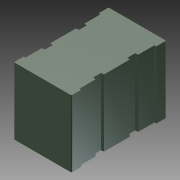
# Autodesk Inventor part: M20111SS1W01-switch
Saved by Autodesk Inventor 2015 SP1 (Build 190203100, 203)
## iProperties
Category: PARTsolutions
Company: NKKSWITCHES
Created: 2013-12-29
Part Number: M20111SS1W01-switch
Catalog Web Link: www.cadenas.de
Description: Bushing Mount Miniature Toggles - Switch-Series M - Miniature Toggles
Vendor: NKKSWITCHES
Document SubType Name: Modeling
Designer: PARTuser1
Manufacturer: NKKSWITCHES
Density: 1 g/cm^3
Material: Generic
Appearance: RGB(78.00000295042994,110.00000104308060,71.00000336766270)
PSOL_IDENT_0: {$CADENAS_DATA\23d-libs\nkkswitches\toggle\m\parts\m_bt_switch.prj},260 {VTYP=3D},{NB=M20111SS1W01-s
PSOL_IDENT_1: witch},{LINA=M20111SS1W01-switch},{NN=Bushing Mount Miniature Toggles - Switch},{DATE=28.05.2013 10:
PSOL_IDENT_2: 56:01},{GEOMDATE=28.05.2013 12:19:00},{VERSION=},{LINEID=10},{LINESUBID=-1},{WBVAR=PLS,CRCTS,TGGL,TG
PSOL_IDENT_3: GLS,BSHNG,CMR,TRMNLS,CPS,CCLR}  {NB=M20111SS1W01-switch},{LINA=M20111SS1W01-switch},{KT=DUMMY},{PN=M
PSOL_IDENT_4: 20111SS1W01},{SRS=M20},{PLS=1},{CRCTSALG='1','1 - ON/NONE/OFF','2','2 - ON/NONE/ON','3','3 - ON/OFF/
PSOL_IDENT_5: ON','5','5 - ON/NONE/(ON)','8','8 - (ON)/OFF/(ON)','9','9 - ON/OFF/(ON)','4', '4 - ON/ON/ON','6','6
PSOL_IDENT_6: - (ON)/ON/(ON)','7','7 - ON/ON/(ON)'},{CRCTS=1},{TGGL=1},{TGGLSALG='S', 'S - .413\" (10.5mm) Bat','S
PSOL_IDENT_7: 2', 'S2 - .200\" (5.08mm) Bat','S3', 'S3 - .256\" (6.5mm) Bat','E', 'E - .450\" (11.4mm) Flatted','E
PSOL_IDENT_8: 2', 'E2 - .256\" (6.5mm) Flatted','E4', 'E4 - .840\" (21.3mm) Flatted','Q', 'Q - .550\" (14.0mm) Con
PSOL_IDENT_9: e','Q2', 'Q2 - .640\" (16.26mm) Cone','Q4', 'Q4 - .840\" (21.3mm) Cone','C', 'C - .571\" (14.5mm) Co
PSOL_IDENT_10: lor Tipped Cone','D', 'D - .840\" (21.3mm) Color Tipped Cone','K1', 'K1 - .370\" (9.4mm) Paddle','K2
PSOL_IDENT_11: ', 'K2 - .559\" (14.2mm) Paddle'},{TGGLS=S},{BSHNGALG='S1', 'S1 - .350\" (8.9mm) Threaded with Keywa
PSOL_IDENT_12: y','S2', 'S2 - .350\" (8.9mm) Smooth with Keyway','A1', 'A1 - .280\" (7.1mm) Threaded with Keyway','
PSOL_IDENT_13: A2', 'A2 - .280\" (7.1mm) Smooth with Keyway','D1', 'D1 - .350\" (8.9mm) Threaded with D Flat','D4'
PSOL_IDENT_14: , 'D4 - 6mm .350\" (8.9mm) Threaded with D Flat ' ,'D3', 'D3 - .350\" (8.9mm) Threaded Splashproof w
PSOL_IDENT_15: ith D Flat','S4', 'S4 - 6mm .350\" (8.9mm) Threaded with Keyway','D8', 'D8 - 6mm .350\" (8.9mm) Thre
PSOL_IDENT_16: aded Splashproof with D Flat'},{BSHNG=S1},{CMR=W},{TRMNLSALG='01','01 - Solder Lug','02','02 - Quick
PSOL_IDENT_17: Connect','03','03 - .250\" (6.35mm) Straight PC','05', '05 - .425\" (10.8mm) Wirewrap','06', '06 -
PSOL_IDENT_18: .750\" (19.05mm) Wirewrap','07', '07 - .964\" (24.5mm) Wirewrap','08', '08 - 1.062\" (27.0mm) Wirewr
PSOL_IDENT_19: ap'},{TRMNLS=01},{CPSALG='','w/o Cap','B', 'B - For S Bat Toggle','C', 'C - Conical Cap for S Bat To
PSOL_IDENT_20: ggle'},{CPS=},{CPSPN=},{CCLRALG='','N/A'},{CCLR=},{DSH=},{WIDTH=0.512},{HEIGHT=0.371},{LENGTH=0.311}
PSOL_IDENT_21: ,{A=0},{TRMNLNOH=1},{ROTALG=0.2625},{ANG=12.5},{TRMNLOV=2},{LTRMNL=0.079},{POS=0}
CNS_NN: Bushing Mount Miniature Toggles - Switch
CNS_NT: Series M - Miniature Toggles
CNS_NB: M20111SS1W01-switch
CNS_NBSYN: $PN.-switch
CNS_LINA: M20111SS1W01-switch
CNS_PN: M20111SS1W01
CNS_SRS: M20
CNS_PLS: 1 - SPST/SPDT
CNS_CRCTSALG: '1','1 - ON/NONE/OFF','2','2 - ON/NONE/ON','3','3 - ON/OFF/ON','5','5 - ON/NONE/(ON)','8','8 - (ON)/OFF/(ON)','9','9 - ON/OFF/(ON)','4', '4 - ON/ON/ON','6','6 - (ON)/ON/(ON)','7','7 - ON/ON/(ON)'
CNS_CRCTS: 1 - ON/NONE/OFF
CNS_TGGL: Small Toggles
CNS_TGGLSALG: 'S', 'S - .413" (10.5mm) Bat','S2', 'S2 - .200" (5.08mm) Bat','S3', 'S3 - .256" (6.5mm) Bat','E', 'E - .450" (11.4mm) Flatted','E2', 'E2 - .256" (6.5mm) Flatted','E4', 'E4 - .840" (21.3mm) Flatted','Q', 'Q - .550" (14.0mm) Cone','Q2', 'Q2 - .640" (16.26mm) Cone','Q4', 'Q4 - .840" (21.3mm) Cone','C', 'C - .571" (14.5mm) Color Tipped Cone','D', 'D - .840" (21.3mm) Color Tipped Cone','K1', 'K1 - .370" (9.4mm) Paddle','K2', 'K2 - .559" (14.2mm) Paddle'
CNS_TGGLS: S - .413" (10.5mm) Bat
CNS_BSHNGALG: 'S1', 'S1 - .350" (8.9mm) Threaded with Keyway','S2', 'S2 - .350" (8.9mm) Smooth with Keyway','A1', 'A1 - .280" (7.1mm) Threaded with Keyway','A2', 'A2 - .280" (7.1mm) Smooth with Keyway','D1', 'D1 - .350" (8.9mm) Threaded with D Flat','D4' , 'D4 - 6mm .350" (8.9mm) Threaded with D Flat ' ,'D3', 'D3 - .350" (8.9mm) Threaded Splashproof with D Flat','S4', 'S4 - 6mm .350" (8.9mm) Threaded with Keyway','D8', 'D8 - 6mm .350" (8.9mm) Threaded Splashproof with D Flat'
CNS_BSHNG: S1 - .350" (8.9mm) Threaded with Keyway
CNS_CMR: W - Silver; Rated 6A @ 125V AC & 3A @ 250V AC
CNS_TRMNLSALG: '01','01 - Solder Lug','02','02 - Quick Connect','03','03 - .250" (6.35mm) Straight PC','05', '05 - .425" (10.8mm) Wirewrap','06', '06 - .750" (19.05mm) Wirewrap','07', '07 - .964" (24.5mm) Wirewrap','08', '08 - 1.062" (27.0mm) Wirewrap'
CNS_TRMNLS: 01 - Solder Lug
CNS_CPSALG: '','w/o Cap','B', 'B - For S Bat Toggle','C', 'C - Conical Cap for S Bat Toggle'
CNS_CPS: w/o Cap
CNS_CCLRALG: '','N/A'
CNS_CCLR: N/A
CNS_WIDTH: 0.512
CNS_HEIGHT: 0.371
CNS_LENGTH: 0.311
CNS_A: 0.000
CNS_TRMNLNOH: 1.000
CNS_ROTALG: 0.262
CNS_ANG: 12.500
CNS_TRMNLOV: 2.000
CNS_LTRMNL: 0.079
CNS_POS: 0.000
SUPPLIER: NKKSWITCHES
ARTICLENO: M20111SS1W01-switch
BOMINFO: M20111SS1W01-switch
CREATOR: CADENAS GmbH
Title: M20111SS1W01-switch
Author: Cadenas PARTsolutions
Comments: Series M - Miniature Toggles
Autodesk Inventor part; units mm, degrees
sketch "Sketch_2" plane through (0, -0.254, 0) normal (0, 1, 0) x (1, 0, 0)
  line L0 (-3.9497, -5.1435) -> (-3.9497, -6.3724)
  arc A0 (-3.9497, -6.3724) -> (-3.8197, -6.5024) centre (-3.8197, -6.3724) ccw
  line L1 (-3.8197, -6.5024) -> (3.8197, -6.5024)
  arc A1 (3.8197, -6.5024) -> (3.9497, -6.3724) centre (3.8197, -6.3724) ccw
  line L2 (3.9497, -6.3724) -> (3.9497, -5.1435)
  line L3 (3.9497, -5.1435) -> (3.6957, -5.1435)
  line L4 (3.6957, -5.1435) -> (3.6957, -2.9397)
  line L5 (3.6957, -2.9397) -> (3.3147, -2.8725)
  line L6 (3.3147, -2.8725) -> (3.3147, -1.8265)
  line L7 (3.3147, -1.8265) -> (3.6957, -1.7593)
  line L8 (3.6957, -1.7593) -> (3.6957, 1.7593)
  line L9 (3.6957, 1.7593) -> (3.3147, 1.8265)
  line L10 (3.3147, 1.8265) -> (3.3147, 2.8725)
  line L11 (3.3147, 2.8725) -> (3.6957, 2.9397)
  line L12 (3.6957, 2.9397) -> (3.6957, 5.1435)
  line L13 (3.6957, 5.1435) -> (3.9497, 5.1435)
  line L14 (3.9497, 5.1435) -> (3.9497, 6.3724)
  arc A2 (3.9497, 6.3724) -> (3.8197, 6.5024) centre (3.8197, 6.3724) ccw
  line L15 (3.8197, 6.5024) -> (-3.8197, 6.5024)
  arc A3 (-3.8197, 6.5024) -> (-3.9497, 6.3724) centre (-3.8197, 6.3724) ccw
  line L16 (-3.9497, 6.3724) -> (-3.9497, 5.1435)
  line L17 (-3.9497, 5.1435) -> (-3.6957, 5.1435)
  line L18 (-3.6957, 5.1435) -> (-3.6957, 2.9397)
  line L19 (-3.6957, 2.9397) -> (-3.3147, 2.8725)
  line L20 (-3.3147, 2.8725) -> (-3.3147, 1.8265)
  line L21 (-3.3147, 1.8265) -> (-3.6957, 1.7593)
  line L22 (-3.6957, 1.7593) -> (-3.6957, -1.7593)
  line L23 (-3.6957, -1.7593) -> (-3.3147, -1.8265)
  line L24 (-3.3147, -1.8265) -> (-3.3147, -2.8725)
  line L25 (-3.3147, -2.8725) -> (-3.6957, -2.9397)
  line L26 (-3.6957, -2.9397) -> (-3.6957, -5.1435)
  line L27 (-3.6957, -5.1435) -> (-3.9497, -5.1435)
  constraints: 56 end point, 8 point on circle, 4 centre point
extrude "Extrusion1" add sketch "Sketch_2" against normal blind 9.1694
sketch "Sketch_1" plane through (0, -9.4234, 0) normal (0, 1, 0) x (1, 0, 0)
  line L0 (-3.1877, 6.1184) -> (-3.1877, -6.1184)
  arc A0 (-3.1877, -6.1184) -> (-3.0577, -6.2484) centre (-3.0577, -6.1184) ccw
  line L1 (-3.0577, -6.2484) -> (3.0577, -6.2484)
  arc A1 (3.0577, -6.2484) -> (3.1877, -6.1184) centre (3.0577, -6.1184) ccw
  line L2 (3.1877, -6.1184) -> (3.1877, 6.1184)
  arc A2 (3.1877, 6.1184) -> (3.0577, 6.2484) centre (3.0577, 6.1184) ccw
  line L3 (3.0577, 6.2484) -> (-3.0577, 6.2484)
  arc A3 (-3.0577, 6.2484) -> (-3.1877, 6.1184) centre (-3.0577, 6.1184) ccw
  constraints: 8 end point, 8 point on circle, 4 centre point
extrude "Extrusion2" cut sketch "Sketch_1" along normal blind 0.0254
sketch "Sketch_7" plane through (0, -9.4234, 0) normal (0, 1, 0) x (1, 0, 0)
  line L0 (-1.0033, 5.0927) -> (-1.0033, 4.3053)
  line L1 (-1.0033, 4.3053) -> (1.0033, 4.3053)
  line L2 (1.0033, 4.3053) -> (1.0033, 5.0927)
  line L3 (1.0033, 5.0927) -> (-1.0033, 5.0927)
  constraints: 8 end point
extrude "Extrusion3" cut sketch "Sketch_7" along normal blind 0.254
pattern_linear "Rectangular Pattern1" count 2 spacing 4.699 along (0, 0, 1) of "Extrusion3"
ref_plane "rot_XY" through (0, 6.6675, 0) normal (1, 0, 0) x (0, 0, -1)
ref_plane "rot_YZ" through (0, 6.6675, 0) normal (0, 0, -1) x (0, 1, 0)
ref_plane "rot_ZX" through (0, 6.6675, 0) normal (0, 1, 0) x (1, 0, 0)
ref_plane "to_cover_XY" through (0, -0.254, 0) normal (0, 1, 0) x (1, 0, 0)
ref_plane "to_cover_YZ" through (0, -0.254, 0) normal (1, 0, 0) x (0, 0, -1)
ref_plane "to_cover_ZX" through (0, -0.254, 0) normal (0, 0, -1) x (0, 1, 0)
ref_plane "to_terminals_XY" through (0, -9.4234, 0) normal (0, 1, 0) x (1, 0, 0)
ref_plane "to_terminals_YZ" through (0, -9.4234, 0) normal (1, 0, 0) x (0, 0, -1)
ref_plane "to_terminals_ZX" through (0, -9.4234, 0) normal (0, 0, -1) x (0, 1, 0)
body "Solid1"
